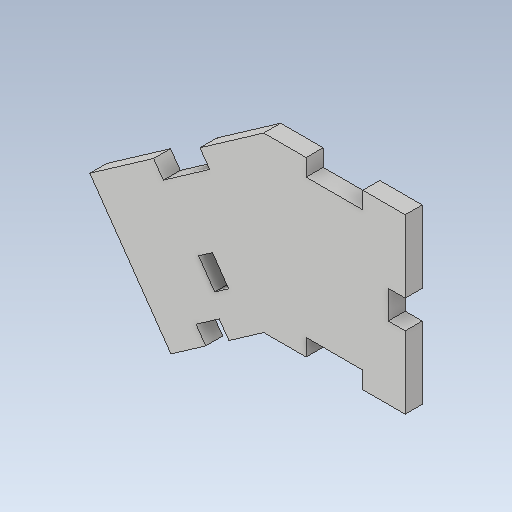
# Autodesk Inventor part: Lateral
Saved by Autodesk Inventor 2020 (Build 240168000, 168)
## iProperties
Created: 2020-03-13
Part Number: Lateral
Material: Genérico
Document SubType Name: Modeling
Designer: joser
Density: 1 g/cm^3
Appearance: Valor por defecto
Author: joser
Autodesk Inventor part; units mm, degrees
ref_plane "YZ Plane" through (0, 0, 0) normal (1, 0, 0) x (0, 1, 0)
ref_plane "XZ Plane" through (0, 0, 0) normal (0, 1, 0) x (-1, 0, 0)
ref_plane "XY Plane" through (0, 0, 0) normal (0, 0, 1) x (1, 0, 0)
sketch "Boceto1" plane through (0, 0, 0) normal (0, 0, 1) x (1, 0, 0)
  line L0 (0, 0) -> (-14.3394, 20.4788)
  line L1 (16.383, 41.9909) -> (16.383, 11.4715)
  line L2 (7.3295, 19.171) -> (10.1973, 15.0753)
  line L3 (10.1973, 15.0753) -> (7.7399, 13.3546)
  line L4 (7.7399, 13.3546) -> (4.872, 17.4503)
  line L5 (4.872, 17.4503) -> (7.3295, 19.171)
  line L6 (23.883, 11.4715) -> (23.883, 14.4715)
  line L7 (23.883, 14.4715) -> (33.883, 14.4715)
  line L8 (33.883, 14.4715) -> (33.883, 11.4715)
  line L9 (41.383, 11.4715) -> (33.883, 11.4715)
  line L10 (23.883, 11.4715) -> (16.383, 11.4715)
  line L11 (41.383, 29.2312) -> (38.383, 29.2312)
  line L12 (38.383, 29.2312) -> (38.383, 24.2312)
  line L13 (38.383, 24.2312) -> (41.383, 24.2312)
  line L14 (41.383, 41.9909) -> (41.383, 29.2312)
  line L15 (41.383, 24.2312) -> (41.383, 11.4715)
  line L16 (23.883, 41.9909) -> (23.883, 38.9909)
  line L17 (23.883, 38.9909) -> (33.883, 38.9909)
  line L18 (33.883, 38.9909) -> (33.883, 41.9909)
  line L19 (16.383, 41.9909) -> (23.883, 41.9909)
  line L20 (33.883, 41.9909) -> (41.383, 41.9909)
  line L21 (-3.0739, 28.367) -> (-1.3532, 25.9095)
  line L22 (-1.3532, 25.9095) -> (6.8383, 31.6453)
  line L23 (6.8383, 31.6453) -> (5.1176, 34.1027)
  line L24 (-14.3394, 20.4788) -> (-3.0739, 28.367)
  line L25 (5.1176, 34.1027) -> (16.383, 41.9909)
  line L26 (6.1436, 4.3018) -> (4.4229, 6.7593)
  line L27 (4.4229, 6.7593) -> (8.5187, 9.6272)
  line L28 (8.5187, 9.6272) -> (10.2394, 7.1697)
  line L29 (16.383, 11.4715) -> (10.2394, 7.1697)
  line L30 (6.1436, 4.3018) -> (0, 0)
  line L31 (16.383, 11.4715) -> (3.7644, 29.4929)
  dimension "d8" = 20
  dimension "d9" = 25
  dimension "d14" = 5
  dimension "d22" = 14
  dimension "d23" = 3
  dimension "d26" = 3
  dimension "d27" = 10
  dimension "d31" = 5
  dimension "d32" = 3
  dimension "d34" = 37.5052
  dimension "d35" = 10
  dimension "d40" = 5
  dimension "d41" = 3
  dimension "d42" = 25
  dimension "d43" = 125
  dimension "d45" = 3
  dimension "d47" = 3.5
  constraints: 65 end point, 32 perpendicular, 10 equal length, 3 horizontal, 3 vertical, 2 collinear, 1 point on line
  measures "d8" distance of L1.end L0.start
  measures "d9" distance of L1.start L14.start
  measures "d14" distance between parallel lines of L3 L5
  measures "d22" distance between parallel lines of L0 L4
  measures "d23" distance between parallel lines of L2 L4
  measures "d26" distance of L6.start L6.end
  measures "d27" distance between parallel lines of L8 L6
  measures "d31" distance of L11.end L12.end
  measures "d32" distance between parallel lines of L14 L12
  measures "d34" distance of L0.end L1.start
  measures "d35" distance between parallel lines of L23 L21
  measures "d40" distance between parallel lines of L28 L26
  measures "d41" distance between parallel lines of L27 L30
  measures "d42" distance between parallel lines of L30 L24
  measures "d43" angle of L29 L1
  measures "d45" distance between parallel lines of L22 L24
  measures "d47" distance between parallel lines of L3 L27
extrude "Extrusión1" add sketch "Boceto1" along normal blind 3
